Autodesk Fusion 360 part; units mm, degrees
(part 3 of 3)
sketch "Sketch8" plane through (0, 0, -71) normal (0, 0, 1) x (-1, 0, 0) in component "DipCase"
  line L0 (23.45, 45.575) -> (23.45, 72.575)
  arc A0 (18.95, 77.075) -> (23.45, 72.575) centre (23.45, 77.075) ccw
  line L1 (18.95, 77.075) -> (-57.05, 77.075)
  arc A1 (-61.55, 72.575) -> (-57.05, 77.075) centre (-61.55, 77.075) ccw
  line L2 (-61.55, 72.575) -> (-61.55, 66.575)
  line L3 (-61.55, 66.575) -> (-62.84, 66.575)
  line L4 (-62.84, 66.575) -> (-62.84, 51.575)
  line L5 (-62.84, 51.575) -> (-61.55, 51.575)
  line L6 (-61.55, 51.575) -> (-61.55, 45.575)
  arc A2 (-57.05, 41.075) -> (-61.55, 45.575) centre (-61.55, 41.075) ccw
  line L7 (-57.05, 41.075) -> (18.95, 41.075)
  arc A3 (23.45, 45.575) -> (18.95, 41.075) centre (23.45, 41.075) ccw
  line L8 (-61.55, 66.575) -> (-61.55, 51.575)
  constraint coincident L2.end L3.start
  constraint coincident L5.end L6.start
extrude "Extrude7''" add sketch "Sketch8" along normal blind 30 contours L3 L4 L5 L8 bodies 5 in component "DipCase"
sketch "Sketch9" plane through (61.55, 0, 0) normal (-1, 0, 0) x (0, -1, 0) in component "DipCase"
  line L0 (45.575, -71) -> (72.575, -71)
  line L1 (72.575, -71) -> (72.575, -5.6)
  line L2 (72.575, -5.6) -> (66.575, -5.6)
  line L3 (66.575, -5.6) -> (66.575, -41)
  line L4 (66.575, -41) -> (51.575, -41)
  line L5 (51.575, -41) -> (51.575, -5.6)
  line L6 (51.575, -5.6) -> (45.575, -5.6)
  line L7 (45.575, -5.6) -> (45.575, -71)
  line L8 (51.575, -41) -> (45.575, -41)
  line L9 (45.575, -41) -> (66.575, -41)
  line L10 (66.575, -41) -> (72.575, -41)
  line L11 (59.075, -41) -> (59.075, -71) construction
  line L12 (48.075, -51) -> (70.075, -51)
  line L13 (70.075, -51) -> (70.075, -61)
  line L14 (70.075, -61) -> (48.075, -61)
  line L15 (48.075, -61) -> (48.075, -51)
  line L16 (48.075, -51) -> (70.075, -61) construction
  line L17 (70.075, -51) -> (48.075, -61) construction
  line L18 (54.075, -54) -> (64.075, -54)
  line L19 (64.075, -54) -> (64.075, -58)
  line L20 (64.075, -58) -> (54.075, -58)
  line L21 (54.075, -58) -> (54.075, -54)
  line L22 (54.075, -54) -> (64.075, -58) construction
  line L23 (64.075, -54) -> (54.075, -58) construction
  point P0 (59.075, -56)
  point P1 (59.075, -56)
  point P2 (59.075, -56)
  dimension "d257" = 22
  dimension "d258" = 10
  dimension "d259" = 10
  dimension "d260" = 4
  constraint coincident L4.end L5.start
  constraint coincident L7 L8.end
  constraint perpendicular L7 L8
  constraint coincident L3.end L4.start
  constraint coincident L1 L10.end
  constraint perpendicular L1 L10
  constraint midpoint L4 L11.start
  constraint midpoint L0 L11.end
  constraint midpoint L11 P2
  constraint horizontal L12
  constraint perpendicular L12 L13
  constraint parallel L12 L14
  constraint parallel L13 L15
  constraint coincident L16 P2
  constraint coincident L17 P2
  constraint coincident P2 P1
  constraint horizontal L18
  constraint perpendicular L18 L19
  constraint parallel L18 L20
  constraint parallel L19 L21
  constraint coincident L22 P2
  constraint coincident L23 P2
  measures "d257" distance of L13.end L14.end
  measures "d258" distance of L12.end L13.end
  measures "d259" distance of L19.end L20.end
  measures "d260" distance of L18.end L19.end
extrude "Extrude8''" cut sketch "Sketch9" against normal up to surface (5 mm away) contours L18 L19 L20 L21 bodies 5 in component "DipCase"
extrude "Extrude9'" cut sketch "Sketch9" against normal blind 3 contours L12 L13 L14 L15 bodies 5 in component "DipCase"
sketch "Sketch10" plane through (0, -82.075, 0) normal (0, -1, 0) x (1, 0, 0) in component "DipCase"
  line L0 (45.85, -44.8) -> (-7.75, -44.8)
  line L1 (-7.75, -44.8) -> (-7.75, -36.2)
  line L2 (-7.75, -36.2) -> (45.85, -36.2)
  line L3 (45.85, -36.2) -> (45.85, -44.8)
  line L4 (-25.45, -76) -> (63.55, -76)
  line L5 (63.55, -76) -> (63.55, -5.6)
  line L6 (63.55, -5.6) -> (-25.45, -5.6)
  line L7 (-25.45, -5.6) -> (-25.45, -76)
  line L8 (42.85, -41.8) -> (-4.75, -41.8)
  line L9 (-4.75, -41.8) -> (-4.75, -39.2)
  line L10 (-4.75, -39.2) -> (42.85, -39.2)
  line L11 (42.85, -39.2) -> (42.85, -41.8)
  dimension "d268" = 3
extrude "Extrude11" add sketch "Sketch10" against normal up to surface (5 mm away) contours L0 L1 L2 L3 bodies 5 in component "DipCase"
component "Plate" placed x (1, 0, 0) y (0, 1, 0) z (0, 0, 1) at (0, 0, 0)
component "Case" placed x (1, 0, 0) y (0, 1, 0) z (0, 0, 1) at (0, 0, 0)
component "DipPlate" placed x (-1, 0, 0) y (0, -1, 0) z (0, 0, 1) at (17.84, -59.075, -5.6)
component "DipCase" placed x (1, 0, 0) y (0, 1, 0) z (0, 0, 1) at (0, 0, 0)
component "Insert" placed x (1, 0, 0) y (0, 1, 0) z (0, 0, 1) at (0, 0, 0) in component "Plate"
equation "WallThickness = 5 mm"
equation "d24 = 80 mm + ( WallThickness * 2 ) + 5 mm"
equation "d25 = WallThickness * 2"
equation "d32 = M3HoleDiameter"
equation "d35 = WallThickness * 2"
equation "d100 = -WallThickness"
equation "M3InsertDiameter = 4.6 mm"
equation "M3InsertLength = 6 mm"
equation "d103 = M3InsertDiameter"
equation "d105 = M3InsertLength"
equation "d109 = WallThickness"
equation "d118 = 68 mm - 2.19 mm"
equation "d119 = 28.18 mm - 2.19 mm"
equation "M1p6InsertDiameter = 2.3 mm"
equation "M1p6InsertLength = 4 mm"
equation "d122 = M1p6InsertDiameter"
equation "d124 = M3InsertLength"
equation "d126 = M1p6InsertLength + 16 mm"
equation "d143 = 68 mm - 2.19 mm"
equation "d144 = 28.18 mm - 2.19 mm"
equation "d145 = M1p6InsertDiameter"
equation "d148 = M1p6InsertDiameter"
equation "d149 = -M1p6InsertLength"
equation "d152 = M3HoleDiameter"
equation "d161 = M1p6InsertDiameter"
equation "d168 = 5.35 mm + 27.94 mm + 0.5 mm"
equation "d173 = 3 mm + WallThickness"
equation "d214 = M1p6InsertLength"
equation "d216 = -WallThickness"
equation "M3HoleDiameter = 4 mm"
equation "d219 = M3HoleDiameter"
equation "d230 = -WallThickness"
equation "d233 = M3InsertDiameter"
equation "d250 = M3InsertDiameter"
equation "d263 = -WallThickness + 2 mm"
equation "d265 = M3InsertLength"
